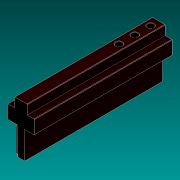
# Autodesk Inventor part: slider
Saved by Autodesk Inventor 2020.3 (Build 243373000, 373)
## iProperties
Created: 2020-05-25
Part Number: slider
Material: Generic
Document SubType Name: Modeling
Designer: Svend
Density: 1 g/cm^3
Appearance: Default
Author: Svend
Autodesk Inventor part; units mm, degrees
(part 1 of 2)
ref_plane "YZ Plane" through (0, 0, 0) normal (1, 0, 0) x (0, 1, 0)
ref_plane "XZ Plane" through (0, 0, 0) normal (0, 1, 0) x (-1, 0, 0)
ref_plane "XY Plane" through (0, 0, 0) normal (0, 0, 1) x (1, 0, 0)
sketch "Sketch1" plane through (0, 0, 0) normal (0, 0, 1) x (1, 0, 0)
  line L0 (-3.25, 4.8) -> (3.25, 4.8)
  line L1 (3.25, 4.8) -> (3.25, 0)
  line L2 (3.25, 0) -> (6.8, 0)
  line L3 (6.8, 0) -> (6.8, -7)
  line L4 (-3, -21) -> (-3, -7)
  line L5 (-6.8, -7) -> (-6.8, 0)
  line L6 (-6.8, 0) -> (-3.25, 0)
  line L7 (-3.25, 4.8) -> (-3.25, 0)
  line L8 (-3, -21) -> (3, -21)
  line L9 (6.8, -7) -> (3, -7)
  line L10 (-6.8, -7) -> (-3, -7)
  line L11 (3, -21) -> (3, -7)
  point P0 (0, 0)
  point P1 (0, 4.8)
  point P2 (0, -17.2)
  point P3 (0, -21)
  dimension "d0" = 6.5
  dimension "d1" = 4.8
  dimension "d6" = 14
  dimension "d7" = 7
  dimension "d8" = 6
  dimension "d9" = 13.6
  constraints: 24 end point, 5 perpendicular, 4 horizontal, 3 equal length, 3 point on line, 3 vertical alignment, 2 midpoint, 2 vertical
  measures "d0" distance between parallel lines of L7 L1
  measures "d1" distance between parallel lines of L2 L0
  measures "d6" distance of L4.start L4.end
  measures "d7" distance of L2.end L3.end
  measures "d8" distance between parallel lines of L4 L11
  measures "d9" distance between parallel lines of L5 L3
extrude "Extrusion1" add sketch "Sketch1" along normal mid plane 70
sketch "Sketch2" plane through (-3.25, 4.8, 35) normal (0, 1, 0) x (1, 0, 0)
  line L0 (0, 70) -> (0, 0) projected
  line L1 (6.5, 0) -> (0, 0) projected
  line L2 (6.5, 70) -> (6.5, 0) projected
  line L3 (0, 70) -> (6.5, 70) projected
  circle A0 centre (3.25, 49.7) radius 1.6
  circle A1 centre (3.25, 57.7) radius 1.6
  circle A2 centre (3.25, 65.7) radius 1.6
  point P0 (3.25, 35)
  dimension "d13" = 4.3
  dimension "d14" = 8
  dimension "d15" = 8
  dimension "d17" = 3.2
  constraints: 3 centre point, 3 coincident, 3 vertical alignment, 2 equal radius
  measures "d13" distance from line of point (3.25, 65.7) L3
  measures "d14" distance of point (3.25, 57.7) point (3.25, 65.7)
  measures "d15" distance of point (3.25, 57.7) point (3.25, 49.7)
  measures "d17" diameter of A0
extrude "Extrusion2" cut sketch "Sketch2" against normal blind 8.3 contours A0 | A1 | A2
sketch "Sketch3" plane through (0, 0, -35) normal (0, 0, -1) x (-1, 0, 0)
  line L0 (3, -21) -> (3, -7) projected
  line L1 (3, -7) -> (6.8, -7) projected
  line L2 (6.8, -7) -> (6.8, 0) projected
  line L3 (6.8, 0) -> (3.25, 0) projected
  line L4 (3.25, 0) -> (3.25, 4.8) projected
  line L5 (3.25, 4.8) -> (-3.25, 4.8) projected
  line L6 (-3.25, 4.8) -> (-3.25, 0) projected
  line L7 (-3.25, 0) -> (-6.8, 0) projected
  line L8 (-6.8, 0) -> (-6.8, -7) projected
  line L9 (-6.8, -7) -> (-3, -7) projected
  line L10 (-3, -7) -> (-3, -21) projected
  line L11 (-3, -21) -> (3, -21) projected
  line L12 (-1.6, -3.5) -> (1.6, -3.5) projected
  line L13 (-2.75, -1.5) -> (2.75, -1.5)
  line L14 (2.75, -1.5) -> (2.75, -5.5)
  line L15 (2.75, -5.5) -> (-2.75, -5.5)
  line L16 (-2.75, -5.5) -> (-2.75, -1.5)
  line L17 (-2.75, -1.5) -> (2.75, -5.5) construction
  line L18 (2.75, -1.5) -> (-2.75, -5.5) construction
  point P0 (0, 0)
  point P1 (0, -3.5)
  dimension "d21" = 5.5
  dimension "d22" = 4
  constraints: 12 end point, 3 midpoint, 2 parallel, 1 horizontal, 1 perpendicular
  measures "d21" distance of L14.end L15.end
  measures "d22" distance of L13.end L14.end
extrude "Extrusion3" cut sketch "Sketch3" against normal blind 25 contours L13 L14 L15 L16
chamfer "Chamfer1" distance 0.2 angle 45 8 edges at (6.8, 0, 0) (6.8, -7, 0) (3.25, 4.8, 0) (-3.25, 4.8, 0) (-6.8, 0, 0) (-6.8, -7, 0) (-3, -21, 0) (3, -21, 0)
chamfer "Chamfer2" distance 0.2 angle 45 3 edges at (-1.6, 4.8, -14.7) (-1.6, 4.8, -22.7) (-1.6, 4.8, -30.7)
chamfer "Chamfer3" distance 0.2 angle 45 16 edges at (4.925, 0, -35) (3.25, 2.3, -35) (0, 4.8, -35) (-3.25, 2.3, -35) (-4.925, 0, -35) (-6.8, -3.5, -35) (-4.8, -7, -35) (-3, -13.9, -35) (3, -13.9, -35) (4.8, -7, -35) (6.8, -3.5, -35) (0, -21, -35) (0, -5.5, -35) (-2.75, -3.5, -35) (0, -1.5, -35) (2.75, -3.5, -35)
sketch "Sketch4" plane through (0, 0, 35) normal (0, 0, 1) x (1, 0, 0)
  line L0 (3, -20.8) -> (2.8, -21) projected
  line L1 (3, -20.8) -> (3, -7) projected
  line L2 (3, -7) -> (6.6, -7) projected
  line L3 (6.8, -6.8) -> (6.6, -7) projected
  line L4 (6.8, -6.8) -> (6.8, -0.2) projected
  line L5 (6.6, 0) -> (6.8, -0.2) projected
  line L6 (6.6, 0) -> (3.25, 0) projected
  line L7 (3.25, 0) -> (3.25, 4.6) projected
  line L8 (3.05, 4.8) -> (3.25, 4.6) projected
  line L9 (3.05, 4.8) -> (-3.05, 4.8) projected
  line L10 (-3.25, 4.6) -> (-3.05, 4.8) projected
  line L11 (-3.25, 4.6) -> (-3.25, 0) projected
  line L12 (-3.25, 0) -> (-6.6, 0) projected
  line L13 (-6.8, -0.2) -> (-6.6, 0) projected
  line L14 (-6.8, -0.2) -> (-6.8, -6.8) projected
  line L15 (-6.6, -7) -> (-6.8, -6.8) projected
  line L16 (-6.6, -7) -> (-3, -7) projected
  line L17 (-3, -7) -> (-3, -20.8) projected
  line L18 (-2.8, -21) -> (-3, -20.8) projected
  line L19 (-2.8, -21) -> (2.8, -21) projected
  line L20 (-3, -7) -> (-1, -7)
  line L21 (-1, -7) -> (-1, -21)
  line L22 (2.8, -21) -> (-2.8, -21) projected
  point P0 (0, 0)
  dimension "d37" = 2
  constraints: 4 end point, 1 horizontal, 1 perpendicular, 1 point on line
  measures "d37" distance between parallel lines of L17 L21
extrude "Extrusion4" cut sketch "Sketch4" against normal through all contours L19 L18 L17 L20 L21
sketch "Sketch5" plane through (2.8, -21, -34.8) normal (0, -1, 0) x (1, 0, 0)
  line L0 (-4.55, 1.057) -> (-4.55, 2.6868)
  line L1 (-4.55, 2.6868) -> (-5.5, 2.6868)
  spline S0 degree 3 poles (-5.5, 2.6868) (-5.5115, 2.6868) (-5.5306, 2.6865) (-5.5581, 2.6853) (-5.5836, 2.6837) (-5.6121, 2.6814) (-5.6435, 2.6782) (-5.6779, 2.674) (-5.7151, 2.6686) (-5.7551, 2.6621) (-5.798, 2.6542) (-5.8437, 2.6449) (-5.8921, 2.6339) (-5.9432, 2.6213) (-5.9969, 2.6069) (-6.0532, 2.5906) (-6.1121, 2.5723) (-6.1734, 2.5518) (-6.2372, 2.5292) (-6.3033, 2.5041) (-6.3716, 2.4767) (-6.4422, 2.4467) (-6.5149, 2.4141) (-6.5897, 2.3787) (-6.6664, 2.3405) (-6.745, 2.2994) (-6.8162, 2.2604) (-6.8611, 2.2348) (-6.8794, 2.2242) knots 0 0 0 0 0.023552 0.038904 0.056302 0.075747 0.097239 0.120778 0.146364 0.173997 0.203676 0.235403 0.269176 0.304996 0.342863 0.382777 0.424738 0.468746 0.5148 0.562902 0.61305 0.665245 0.719487 0.775776 0.834112 0.894494 0.956924 1 1 1 1
  arc A0 (-6.8794, 2.2242) -> (-6.8794, 1.5196) centre (2.0124, 1.8719) ccw
  spline S1 degree 3 poles (-6.8794, 1.5196) (-6.8611, 1.509) (-6.8428, 1.4985) (-6.8244, 1.4882) (-6.7977, 1.4733) (-6.7709, 1.4585) (-6.744, 1.4441) (-6.7179, 1.4302) (-6.6917, 1.4165) (-6.6654, 1.403) (-6.6399, 1.39) (-6.6144, 1.3773) (-6.5887, 1.3649) (-6.5639, 1.3528) (-6.5389, 1.341) (-6.5139, 1.3295) (-6.4898, 1.3184) (-6.4655, 1.3075) (-6.4412, 1.2969) (-6.4178, 1.2867) (-6.3942, 1.2767) (-6.3706, 1.2669) (-6.3479, 1.2575) (-6.3251, 1.2484) (-6.3022, 1.2395) (-6.2803, 1.2309) (-6.2583, 1.2226) (-6.2362, 1.2145) (-6.215, 1.2067) (-6.1937, 1.1991) (-6.1724, 1.1918) (-6.152, 1.1848) (-6.1316, 1.178) (-6.1111, 1.1714) (-6.0915, 1.1651) (-6.0719, 1.1589) (-6.0522, 1.153) (-6.0335, 1.1474) (-6.0147, 1.142) (-5.9959, 1.1367) (-5.978, 1.1318) (-5.9601, 1.127) (-5.9422, 1.1224) (-5.9252, 1.118) (-5.9081, 1.1138) (-5.8911, 1.1098) (-5.875, 1.106) (-5.8588, 1.1023) (-5.8427, 1.0988) (-5.8275, 1.0956) (-5.8123, 1.0925) (-5.797, 1.0895) (-5.7827, 1.0867) (-5.7684, 1.0841) (-5.7541, 1.0816) (-5.7408, 1.0793) (-5.7274, 1.0771) (-5.7141, 1.0751) (-5.7017, 1.0732) (-5.6893, 1.0714) (-5.6768, 1.0698) (-5.6654, 1.0683) (-5.654, 1.0669) (-5.6425, 1.0656) (-5.6321, 1.0644) (-5.6216, 1.0633) (-5.6111, 1.0624) (-5.6016, 1.0615) (-5.5921, 1.0607) (-5.5826, 1.06) (-5.5741, 1.0594) (-5.5656, 1.0589) (-5.5571, 1.0585) (-5.5496, 1.0581) (-5.5421, 1.0578) (-5.5346, 1.0575) (-5.5231, 1.0572) (-5.5115, 1.057) (-5.5, 1.057) knots 0 0 0 0 0.043076 0.043076 0.043076 0.105506 0.105506 0.105506 0.165888 0.165888 0.165888 0.224224 0.224224 0.224224 0.280513 0.280513 0.280513 0.334755 0.334755 0.334755 0.38695 0.38695 0.38695 0.437099 0.437099 0.437099 0.4852 0.4852 0.4852 0.531254 0.531254 0.531254 0.575262 0.575262 0.575262 0.617223 0.617223 0.617223 0.657137 0.657137 0.657137 0.695004 0.695004 0.695004 0.730824 0.730824 0.730824 0.764598 0.764598 0.764598 0.796324 0.796324 0.796324 0.826004 0.826004 0.826004 0.853636 0.853636 0.853636 0.879222 0.879222 0.879222 0.902761 0.902761 0.902761 0.924253 0.924253 0.924253 0.943699 0.943699 0.943699 0.961097 0.961097 0.961097 0.976448 0.976448 0.976448 1 1 1 1
  line L2 (-5.5, 1.057) -> (-4.55, 1.057)
  line L3 (-4.55, 4.193) -> (-4.55, 5.8228)
  line L4 (-4.55, 5.8228) -> (-5.5, 5.8228)
  spline S2 degree 3 poles (-5.5, 5.8228) (-5.5115, 5.8228) (-5.5306, 5.8225) (-5.5581, 5.8213) (-5.5836, 5.8197) (-5.6121, 5.8174) (-5.6435, 5.8142) (-5.6779, 5.81) (-5.7151, 5.8046) (-5.7551, 5.7981) (-5.798, 5.7902) (-5.8437, 5.7809) (-5.8921, 5.7699) (-5.9432, 5.7573) (-5.9969, 5.7429) (-6.0532, 5.7266) (-6.1121, 5.7083) (-6.1734, 5.6878) (-6.2372, 5.6652) (-6.3033, 5.6401) (-6.3716, 5.6127) (-6.4422, 5.5827) (-6.5149, 5.5501) (-6.5897, 5.5147) (-6.6664, 5.4765) (-6.745, 5.4354) (-6.8162, 5.3964) (-6.8611, 5.3708) (-6.8794, 5.3602) knots 0 0 0 0 0.023552 0.038904 0.056302 0.075747 0.097239 0.120778 0.146364 0.173997 0.203676 0.235403 0.269176 0.304996 0.342863 0.382777 0.424738 0.468746 0.5148 0.562902 0.61305 0.665245 0.719487 0.775776 0.834112 0.894494 0.956924 1 1 1 1
  arc A1 (-6.8794, 5.3602) -> (-6.8794, 4.6556) centre (2.0124, 5.0079) ccw
  spline S3 degree 3 poles (-6.8794, 4.6556) (-6.8611, 4.645) (-6.8428, 4.6345) (-6.8244, 4.6242) (-6.7977, 4.6093) (-6.7709, 4.5945) (-6.744, 4.5801) (-6.7179, 4.5662) (-6.6917, 4.5525) (-6.6654, 4.539) (-6.6399, 4.526) (-6.6144, 4.5133) (-6.5887, 4.5009) (-6.5639, 4.4888) (-6.5389, 4.477) (-6.5139, 4.4655) (-6.4898, 4.4544) (-6.4655, 4.4435) (-6.4412, 4.4329) (-6.4178, 4.4227) (-6.3942, 4.4127) (-6.3706, 4.4029) (-6.3479, 4.3935) (-6.3251, 4.3844) (-6.3022, 4.3755) (-6.2803, 4.3669) (-6.2583, 4.3586) (-6.2362, 4.3505) (-6.215, 4.3427) (-6.1937, 4.3351) (-6.1724, 4.3278) (-6.152, 4.3208) (-6.1316, 4.314) (-6.1111, 4.3074) (-6.0915, 4.3011) (-6.0719, 4.2949) (-6.0522, 4.289) (-6.0335, 4.2834) (-6.0147, 4.278) (-5.9959, 4.2727) (-5.978, 4.2678) (-5.9601, 4.263) (-5.9422, 4.2584) (-5.9252, 4.254) (-5.9081, 4.2498) (-5.8911, 4.2458) (-5.875, 4.242) (-5.8588, 4.2383) (-5.8427, 4.2348) (-5.8275, 4.2316) (-5.8123, 4.2285) (-5.797, 4.2255) (-5.7827, 4.2227) (-5.7684, 4.2201) (-5.7541, 4.2176) (-5.7408, 4.2153) (-5.7274, 4.2131) (-5.7141, 4.2111) (-5.7017, 4.2092) (-5.6893, 4.2074) (-5.6768, 4.2058) (-5.6654, 4.2043) (-5.654, 4.2029) (-5.6425, 4.2016) (-5.6321, 4.2004) (-5.6216, 4.1993) (-5.6111, 4.1984) (-5.6016, 4.1975) (-5.5921, 4.1967) (-5.5826, 4.196) (-5.5741, 4.1954) (-5.5656, 4.1949) (-5.5571, 4.1945) (-5.5496, 4.1941) (-5.5421, 4.1938) (-5.5346, 4.1935) (-5.5231, 4.1932) (-5.5115, 4.193) (-5.5, 4.193) knots 0 0 0 0 0.043076 0.043076 0.043076 0.105506 0.105506 0.105506 0.165888 0.165888 0.165888 0.224224 0.224224 0.224224 0.280513 0.280513 0.280513 0.334755 0.334755 0.334755 0.38695 0.38695 0.38695 0.437099 0.437099 0.437099 0.4852 0.4852 0.4852 0.531254 0.531254 0.531254 0.575262 0.575262 0.575262 0.617223 0.617223 0.617223 0.657137 0.657137 0.657137 0.695004 0.695004 0.695004 0.730824 0.730824 0.730824 0.764598 0.764598 0.764598 0.796324 0.796324 0.796324 0.826004 0.826004 0.826004 0.853636 0.853636 0.853636 0.879222 0.879222 0.879222 0.902761 0.902761 0.902761 0.924253 0.924253 0.924253 0.943699 0.943699 0.943699 0.961097 0.961097 0.961097 0.976448 0.976448 0.976448 1 1 1 1
  line L5 (-5.5, 4.193) -> (-4.55, 4.193)
  line L6 (-4.55, 7.329) -> (-4.55, 8.9588)
  line L7 (-4.55, 8.9588) -> (-5.5, 8.9588)
  spline S4 degree 3 poles (-5.5, 8.9588) (-5.5115, 8.9588) (-5.5306, 8.9585) (-5.5581, 8.9573) (-5.5836, 8.9557) (-5.6121, 8.9534) (-5.6435, 8.9502) (-5.6779, 8.946) (-5.7151, 8.9406) (-5.7551, 8.9341) (-5.798, 8.9262) (-5.8437, 8.9169) (-5.8921, 8.9059) (-5.9432, 8.8933) (-5.9969, 8.8789) (-6.0532, 8.8626) (-6.1121, 8.8443) (-6.1734, 8.8238) (-6.2372, 8.8012) (-6.3033, 8.7761) (-6.3716, 8.7487) (-6.4422, 8.7187) (-6.5149, 8.6861) (-6.5897, 8.6507) (-6.6664, 8.6125) (-6.745, 8.5714) (-6.8162, 8.5324) (-6.8611, 8.5068) (-6.8794, 8.4962) knots 0 0 0 0 0.023552 0.038904 0.056302 0.075747 0.097239 0.120778 0.146364 0.173997 0.203676 0.235403 0.269176 0.304996 0.342863 0.382777 0.424738 0.468746 0.5148 0.562902 0.61305 0.665245 0.719487 0.775776 0.834112 0.894494 0.956924 1 1 1 1
  arc A2 (-6.8794, 8.4962) -> (-6.8794, 7.7916) centre (2.0124, 8.1439) ccw
  spline S5 degree 3 poles (-6.8794, 7.7916) (-6.8611, 7.781) (-6.8428, 7.7705) (-6.8244, 7.7602) (-6.7977, 7.7453) (-6.7709, 7.7305) (-6.744, 7.7161) (-6.7179, 7.7022) (-6.6917, 7.6885) (-6.6654, 7.675) (-6.6399, 7.662) (-6.6144, 7.6493) (-6.5887, 7.6369) (-6.5639, 7.6248) (-6.5389, 7.613) (-6.5139, 7.6015) (-6.4898, 7.5904) (-6.4655, 7.5795) (-6.4412, 7.5689) (-6.4178, 7.5587) (-6.3942, 7.5487) (-6.3706, 7.5389) (-6.3479, 7.5295) (-6.3251, 7.5204) (-6.3022, 7.5115) (-6.2803, 7.5029) (-6.2583, 7.4946) (-6.2362, 7.4865) (-6.215, 7.4787) (-6.1937, 7.4711) (-6.1724, 7.4638) (-6.152, 7.4568) (-6.1316, 7.45) (-6.1111, 7.4434) (-6.0915, 7.4371) (-6.0719, 7.4309) (-6.0522, 7.425) (-6.0335, 7.4194) (-6.0147, 7.414) (-5.9959, 7.4087) (-5.978, 7.4038) (-5.9601, 7.399) (-5.9422, 7.3944) (-5.9252, 7.39) (-5.9081, 7.3858) (-5.8911, 7.3818) (-5.875, 7.378) (-5.8588, 7.3743) (-5.8427, 7.3708) (-5.8275, 7.3676) (-5.8123, 7.3645) (-5.797, 7.3615) (-5.7827, 7.3587) (-5.7684, 7.3561) (-5.7541, 7.3536) (-5.7408, 7.3513) (-5.7274, 7.3491) (-5.7141, 7.3471) (-5.7017, 7.3452) (-5.6893, 7.3434) (-5.6768, 7.3418) (-5.6654, 7.3403) (-5.654, 7.3389) (-5.6425, 7.3376) (-5.6321, 7.3364) (-5.6216, 7.3353) (-5.6111, 7.3344) (-5.6016, 7.3335) (-5.5921, 7.3327) (-5.5826, 7.332) (-5.5741, 7.3314) (-5.5656, 7.3309) (-5.5571, 7.3305) (-5.5496, 7.3301) (-5.5421, 7.3298) (-5.5346, 7.3295) (-5.5231, 7.3292) (-5.5115, 7.329) (-5.5, 7.329) knots 0 0 0 0 0.043076 0.043076 0.043076 0.105506 0.105506 0.105506 0.165888 0.165888 0.165888 0.224224 0.224224 0.224224 0.280513 0.280513 0.280513 0.334755 0.334755 0.334755 0.38695 0.38695 0.38695 0.437099 0.437099 0.437099 0.4852 0.4852 0.4852 0.531254 0.531254 0.531254 0.575262 0.575262 0.575262 0.617223 0.617223 0.617223 0.657137 0.657137 0.657137 0.695004 0.695004 0.695004 0.730824 0.730824 0.730824 0.764598 0.764598 0.764598 0.796324 0.796324 0.796324 0.826004 0.826004 0.826004 0.853636 0.853636 0.853636 0.879222 0.879222 0.879222 0.902761 0.902761 0.902761 0.924253 0.924253 0.924253 0.943699 0.943699 0.943699 0.961097 0.961097 0.961097 0.976448 0.976448 0.976448 1 1 1 1
  line L8 (-5.5, 7.329) -> (-4.55, 7.329)
  line L9 (-4.55, 10.465) -> (-4.55, 12.0948)
  line L10 (-4.55, 12.0948) -> (-5.5, 12.0948)
  spline S6 degree 3 poles (-5.5, 12.0948) (-5.5115, 12.0948) (-5.5306, 12.0945) (-5.5581, 12.0933) (-5.5836, 12.0917) (-5.6121, 12.0894) (-5.6435, 12.0862) (-5.6779, 12.082) (-5.7151, 12.0766) (-5.7551, 12.0701) (-5.798, 12.0622) (-5.8437, 12.0529) (-5.8921, 12.0419) (-5.9432, 12.0293) (-5.9969, 12.0149) (-6.0532, 11.9986) (-6.1121, 11.9803) (-6.1734, 11.9598) (-6.2372, 11.9372) (-6.3033, 11.9121) (-6.3716, 11.8847) (-6.4422, 11.8547) (-6.5149, 11.8221) (-6.5897, 11.7867) (-6.6664, 11.7485) (-6.745, 11.7074) (-6.8162, 11.6684) (-6.8611, 11.6428) (-6.8794, 11.6322) knots 0 0 0 0 0.023552 0.038904 0.056302 0.075747 0.097239 0.120778 0.146364 0.173997 0.203676 0.235403 0.269176 0.304996 0.342863 0.382777 0.424738 0.468746 0.5148 0.562902 0.61305 0.665245 0.719487 0.775776 0.834112 0.894494 0.956924 1 1 1 1
  arc A3 (-6.8794, 11.6322) -> (-6.8794, 10.9276) centre (2.0124, 11.2799) ccw
  spline S7 degree 3 poles (-6.8794, 10.9276) (-6.8611, 10.917) (-6.8428, 10.9065) (-6.8244, 10.8962) (-6.7977, 10.8813) (-6.7709, 10.8665) (-6.744, 10.8521) (-6.7179, 10.8382) (-6.6917, 10.8245) (-6.6654, 10.811) (-6.6399, 10.798) (-6.6144, 10.7853) (-6.5887, 10.7729) (-6.5639, 10.7608) (-6.5389, 10.749) (-6.5139, 10.7375) (-6.4898, 10.7264) (-6.4655, 10.7155) (-6.4412, 10.7049) (-6.4178, 10.6947) (-6.3942, 10.6847) (-6.3706, 10.6749) (-6.3479, 10.6655) (-6.3251, 10.6564) (-6.3022, 10.6475) (-6.2803, 10.6389) (-6.2583, 10.6306) (-6.2362, 10.6225) (-6.215, 10.6147) (-6.1937, 10.6071) (-6.1724, 10.5998) (-6.152, 10.5928) (-6.1316, 10.586) (-6.1111, 10.5794) (-6.0915, 10.5731) (-6.0719, 10.5669) (-6.0522, 10.561) (-6.0335, 10.5554) (-6.0147, 10.55) (-5.9959, 10.5447) (-5.978, 10.5398) (-5.9601, 10.535) (-5.9422, 10.5304) (-5.9252, 10.526) (-5.9081, 10.5218) (-5.8911, 10.5178) (-5.875, 10.514) (-5.8588, 10.5103) (-5.8427, 10.5068) (-5.8275, 10.5036) (-5.8123, 10.5005) (-5.797, 10.4975) (-5.7827, 10.4947) (-5.7684, 10.4921) (-5.7541, 10.4896) (-5.7408, 10.4873) (-5.7274, 10.4851) (-5.7141, 10.4831) (-5.7017, 10.4812) (-5.6893, 10.4794) (-5.6768, 10.4778) (-5.6654, 10.4763) (-5.654, 10.4749) (-5.6425, 10.4736) (-5.6321, 10.4724) (-5.6216, 10.4713) (-5.6111, 10.4704) (-5.6016, 10.4695) (-5.5921, 10.4687) (-5.5826, 10.468) (-5.5741, 10.4674) (-5.5656, 10.4669) (-5.5571, 10.4665) (-5.5496, 10.4661) (-5.5421, 10.4658) (-5.5346, 10.4655) (-5.5231, 10.4652) (-5.5115, 10.465) (-5.5, 10.465) knots 0 0 0 0 0.043076 0.043076 0.043076 0.105506 0.105506 0.105506 0.165888 0.165888 0.165888 0.224224 0.224224 0.224224 0.280513 0.280513 0.280513 0.334755 0.334755 0.334755 0.38695 0.38695 0.38695 0.437099 0.437099 0.437099 0.4852 0.4852 0.4852 0.531254 0.531254 0.531254 0.575262 0.575262 0.575262 0.617223 0.617223 0.617223 0.657137 0.657137 0.657137 0.695004 0.695004 0.695004 0.730824 0.730824 0.730824 0.764598 0.764598 0.764598 0.796324 0.796324 0.796324 0.826004 0.826004 0.826004 0.853636 0.853636 0.853636 0.879222 0.879222 0.879222 0.902761 0.902761 0.902761 0.924253 0.924253 0.924253 0.943699 0.943699 0.943699 0.961097 0.961097 0.961097 0.976448 0.976448 0.976448 1 1 1 1
  line L11 (-5.5, 10.465) -> (-4.55, 10.465)
  line L12 (-4.55, 13.601) -> (-4.55, 15.2308)
  line L13 (-4.55, 15.2308) -> (-5.5, 15.2308)
  spline S8 degree 3 poles (-5.5, 15.2308) (-5.5115, 15.2308) (-5.5306, 15.2305) (-5.5581, 15.2293) (-5.5836, 15.2277) (-5.6121, 15.2254) (-5.6435, 15.2222) (-5.6779, 15.218) (-5.7151, 15.2126) (-5.7551, 15.2061) (-5.798, 15.1982) (-5.8437, 15.1889) (-5.8921, 15.1779) (-5.9432, 15.1653) (-5.9969, 15.1509) (-6.0532, 15.1346) (-6.1121, 15.1163) (-6.1734, 15.0958) (-6.2372, 15.0732) (-6.3033, 15.0481) (-6.3716, 15.0207) (-6.4422, 14.9907) (-6.5149, 14.9581) (-6.5897, 14.9227) (-6.6664, 14.8845) (-6.745, 14.8434) (-6.8162, 14.8044) (-6.8611, 14.7788) (-6.8794, 14.7682) knots 0 0 0 0 0.023552 0.038904 0.056302 0.075747 0.097239 0.120778 0.146364 0.173997 0.203676 0.235403 0.269176 0.304996 0.342863 0.382777 0.424738 0.468746 0.5148 0.562902 0.61305 0.665245 0.719487 0.775776 0.834112 0.894494 0.956924 1 1 1 1
  arc A4 (-6.8794, 14.7682) -> (-6.8794, 14.0636) centre (2.0124, 14.4159) ccw
  spline S9 degree 3 poles (-6.8794, 14.0636) (-6.8611, 14.053) (-6.8428, 14.0425) (-6.8244, 14.0322) (-6.7977, 14.0173) (-6.7709, 14.0025) (-6.744, 13.9881) (-6.7179, 13.9742) (-6.6917, 13.9605) (-6.6654, 13.947) (-6.6399, 13.934) (-6.6144, 13.9213) (-6.5887, 13.9089) (-6.5639, 13.8968) (-6.5389, 13.885) (-6.5139, 13.8735) (-6.4898, 13.8624) (-6.4655, 13.8515) (-6.4412, 13.8409) (-6.4178, 13.8307) (-6.3942, 13.8207) (-6.3706, 13.8109) (-6.3479, 13.8015) (-6.3251, 13.7924) (-6.3022, 13.7835) (-6.2803, 13.7749) (-6.2583, 13.7666) (-6.2362, 13.7585) (-6.215, 13.7507) (-6.1937, 13.7431) (-6.1724, 13.7358) (-6.152, 13.7288) (-6.1316, 13.722) (-6.1111, 13.7154) (-6.0915, 13.7091) (-6.0719, 13.7029) (-6.0522, 13.697) (-6.0335, 13.6914) (-6.0147, 13.686) (-5.9959, 13.6807) (-5.978, 13.6758) (-5.9601, 13.671) (-5.9422, 13.6664) (-5.9252, 13.662) (-5.9081, 13.6578) (-5.8911, 13.6538) (-5.875, 13.65) (-5.8588, 13.6463) (-5.8427, 13.6428) (-5.8275, 13.6396) (-5.8123, 13.6365) (-5.797, 13.6335) (-5.7827, 13.6307) (-5.7684, 13.6281) (-5.7541, 13.6256) (-5.7408, 13.6233) (-5.7274, 13.6211) (-5.7141, 13.6191) (-5.7017, 13.6172) (-5.6893, 13.6154) (-5.6768, 13.6138) (-5.6654, 13.6123) (-5.654, 13.6109) (-5.6425, 13.6096) (-5.6321, 13.6084) (-5.6216, 13.6073) (-5.6111, 13.6064) (-5.6016, 13.6055) (-5.5921, 13.6047) (-5.5826, 13.604) (-5.5741, 13.6034) (-5.5656, 13.6029) (-5.5571, 13.6025) (-5.5496, 13.6021) (-5.5421, 13.6018) (-5.5346, 13.6015) (-5.5231, 13.6012) (-5.5115, 13.601) (-5.5, 13.601) knots 0 0 0 0 0.043076 0.043076 0.043076 0.105506 0.105506 0.105506 0.165888 0.165888 0.165888 0.224224 0.224224 0.224224 0.280513 0.280513 0.280513 0.334755 0.334755 0.334755 0.38695 0.38695 0.38695 0.437099 0.437099 0.437099 0.4852 0.4852 0.4852 0.531254 0.531254 0.531254 0.575262 0.575262 0.575262 0.617223 0.617223 0.617223 0.657137 0.657137 0.657137 0.695004 0.695004 0.695004 0.730824 0.730824 0.730824 0.764598 0.764598 0.764598 0.796324 0.796324 0.796324 0.826004 0.826004 0.826004 0.853636 0.853636 0.853636 0.879222 0.879222 0.879222 0.902761 0.902761 0.902761 0.924253 0.924253 0.924253 0.943699 0.943699 0.943699 0.961097 0.961097 0.961097 0.976448 0.976448 0.976448 1 1 1 1
  line L14 (-5.5, 13.601) -> (-4.55, 13.601)
  line L15 (-4.55, 16.737) -> (-4.55, 18.3668)
  line L16 (-4.55, 18.3668) -> (-5.5, 18.3668)
  spline S10 degree 3 poles (-5.5, 18.3668) (-5.5115, 18.3668) (-5.5306, 18.3665) (-5.5581, 18.3653) (-5.5836, 18.3637) (-5.6121, 18.3614) (-5.6435, 18.3582) (-5.6779, 18.354) (-5.7151, 18.3486) (-5.7551, 18.3421) (-5.798, 18.3342) (-5.8437, 18.3249) (-5.8921, 18.3139) (-5.9432, 18.3013) (-5.9969, 18.2869) (-6.0532, 18.2706) (-6.1121, 18.2523) (-6.1734, 18.2318) (-6.2372, 18.2092) (-6.3033, 18.1841) (-6.3716, 18.1567) (-6.4422, 18.1267) (-6.5149, 18.0941) (-6.5897, 18.0587) (-6.6664, 18.0205) (-6.745, 17.9794) (-6.8162, 17.9404) (-6.8611, 17.9148) (-6.8794, 17.9042) knots 0 0 0 0 0.023552 0.038904 0.056302 0.075747 0.097239 0.120778 0.146364 0.173997 0.203676 0.235403 0.269176 0.304996 0.342863 0.382777 0.424738 0.468746 0.5148 0.562902 0.61305 0.665245 0.719487 0.775776 0.834112 0.894494 0.956924 1 1 1 1
  arc A5 (-6.8794, 17.9042) -> (-6.8794, 17.1996) centre (2.0124, 17.5519) ccw
  spline S11 degree 3 poles (-6.8794, 17.1996) (-6.8611, 17.189) (-6.8428, 17.1785) (-6.8244, 17.1682) (-6.7977, 17.1533) (-6.7709, 17.1385) (-6.744, 17.1241) (-6.7179, 17.1102) (-6.6917, 17.0965) (-6.6654, 17.083) (-6.6399, 17.07) (-6.6144, 17.0573) (-6.5887, 17.0449) (-6.5639, 17.0328) (-6.5389, 17.021) (-6.5139, 17.0095) (-6.4898, 16.9984) (-6.4655, 16.9875) (-6.4412, 16.9769) (-6.4178, 16.9667) (-6.3942, 16.9567) (-6.3706, 16.9469) (-6.3479, 16.9375) (-6.3251, 16.9284) (-6.3022, 16.9195) (-6.2803, 16.9109) (-6.2583, 16.9026) (-6.2362, 16.8945) (-6.215, 16.8867) (-6.1937, 16.8791) (-6.1724, 16.8718) (-6.152, 16.8648) (-6.1316, 16.858) (-6.1111, 16.8514) (-6.0915, 16.8451) (-6.0719, 16.8389) (-6.0522, 16.833) (-6.0335, 16.8274) (-6.0147, 16.822) (-5.9959, 16.8167) (-5.978, 16.8118) (-5.9601, 16.807) (-5.9422, 16.8024) (-5.9252, 16.798) (-5.9081, 16.7938) (-5.8911, 16.7898) (-5.875, 16.786) (-5.8588, 16.7823) (-5.8427, 16.7788) (-5.8275, 16.7756) (-5.8123, 16.7725) (-5.797, 16.7695) (-5.7827, 16.7667) (-5.7684, 16.7641) (-5.7541, 16.7616) (-5.7408, 16.7593) (-5.7274, 16.7571) (-5.7141, 16.7551) (-5.7017, 16.7532) (-5.6893, 16.7514) (-5.6768, 16.7498) (-5.6654, 16.7483) (-5.654, 16.7469) (-5.6425, 16.7456) (-5.6321, 16.7444) (-5.6216, 16.7433) (-5.6111, 16.7424) (-5.6016, 16.7415) (-5.5921, 16.7407) (-5.5826, 16.74) (-5.5741, 16.7394) (-5.5656, 16.7389) (-5.5571, 16.7385) (-5.5496, 16.7381) (-5.5421, 16.7378) (-5.5346, 16.7375) (-5.5231, 16.7372) (-5.5115, 16.737) (-5.5, 16.737) knots 0 0 0 0 0.043076 0.043076 0.043076 0.105506 0.105506 0.105506 0.165888 0.165888 0.165888 0.224224 0.224224 0.224224 0.280513 0.280513 0.280513 0.334755 0.334755 0.334755 0.38695 0.38695 0.38695 0.437099 0.437099 0.437099 0.4852 0.4852 0.4852 0.531254 0.531254 0.531254 0.575262 0.575262 0.575262 0.617223 0.617223 0.617223 0.657137 0.657137 0.657137 0.695004 0.695004 0.695004 0.730824 0.730824 0.730824 0.764598 0.764598 0.764598 0.796324 0.796324 0.796324 0.826004 0.826004 0.826004 0.853636 0.853636 0.853636 0.879222 0.879222 0.879222 0.902761 0.902761 0.902761 0.924253 0.924253 0.924253 0.943699 0.943699 0.943699 0.961097 0.961097 0.961097 0.976448 0.976448 0.976448 1 1 1 1
  line L17 (-5.5, 16.737) -> (-4.55, 16.737)
  line L18 (-4.55, 19.873) -> (-4.55, 21.5028)
  line L19 (-4.55, 21.5028) -> (-5.5, 21.5028)
  spline S12 degree 3 poles (-5.5, 21.5028) (-5.5115, 21.5028) (-5.5306, 21.5025) (-5.5581, 21.5013) (-5.5836, 21.4997) (-5.6121, 21.4974) (-5.6435, 21.4942) (-5.6779, 21.49) (-5.7151, 21.4846) (-5.7551, 21.4781) (-5.798, 21.4702) (-5.8437, 21.4609) (-5.8921, 21.4499) (-5.9432, 21.4373) (-5.9969, 21.4229) (-6.0532, 21.4066) (-6.1121, 21.3883) (-6.1734, 21.3678) (-6.2372, 21.3452) (-6.3033, 21.3201) (-6.3716, 21.2927) (-6.4422, 21.2627) (-6.5149, 21.2301) (-6.5897, 21.1947) (-6.6664, 21.1565) (-6.745, 21.1154) (-6.8162, 21.0764) (-6.8611, 21.0508) (-6.8794, 21.0402) knots 0 0 0 0 0.023552 0.038904 0.056302 0.075747 0.097239 0.120778 0.146364 0.173997 0.203676 0.235403 0.269176 0.304996 0.342863 0.382777 0.424738 0.468746 0.5148 0.562902 0.61305 0.665245 0.719487 0.775776 0.834112 0.894494 0.956924 1 1 1 1
  arc A6 (-6.8794, 21.0402) -> (-6.8794, 20.3356) centre (2.0124, 20.6879) ccw
  spline S13 degree 3 poles (-6.8794, 20.3356) (-6.8611, 20.325) (-6.8428, 20.3145) (-6.8244, 20.3042) (-6.7977, 20.2893) (-6.7709, 20.2745) (-6.744, 20.2601) (-6.7179, 20.2462) (-6.6917, 20.2325) (-6.6654, 20.219) (-6.6399, 20.206) (-6.6144, 20.1933) (-6.5887, 20.1809) (-6.5639, 20.1688) (-6.5389, 20.157) (-6.5139, 20.1455) (-6.4898, 20.1344) (-6.4655, 20.1235) (-6.4412, 20.1129) (-6.4178, 20.1027) (-6.3942, 20.0927) (-6.3706, 20.0829) (-6.3479, 20.0735) (-6.3251, 20.0644) (-6.3022, 20.0555) (-6.2803, 20.0469) (-6.2583, 20.0386) (-6.2362, 20.0305) (-6.215, 20.0227) (-6.1937, 20.0151) (-6.1724, 20.0078) (-6.152, 20.0008) (-6.1316, 19.994) (-6.1111, 19.9874) (-6.0915, 19.9811) (-6.0719, 19.9749) (-6.0522, 19.969) (-6.0335, 19.9634) (-6.0147, 19.958) (-5.9959, 19.9527) (-5.978, 19.9478) (-5.9601, 19.943) (-5.9422, 19.9384) (-5.9252, 19.934) (-5.9081, 19.9298) (-5.8911, 19.9258) (-5.875, 19.922) (-5.8588, 19.9183) (-5.8427, 19.9148) (-5.8275, 19.9116) (-5.8123, 19.9085) (-5.797, 19.9055) (-5.7827, 19.9027) (-5.7684, 19.9001) (-5.7541, 19.8976) (-5.7408, 19.8953) (-5.7274, 19.8931) (-5.7141, 19.8911) (-5.7017, 19.8892) (-5.6893, 19.8874) (-5.6768, 19.8858) (-5.6654, 19.8843) (-5.654, 19.8829) (-5.6425, 19.8816) (-5.6321, 19.8804) (-5.6216, 19.8793) (-5.6111, 19.8784) (-5.6016, 19.8775) (-5.5921, 19.8767) (-5.5826, 19.876) (-5.5741, 19.8754) (-5.5656, 19.8749) (-5.5571, 19.8745) (-5.5496, 19.8741) (-5.5421, 19.8738) (-5.5346, 19.8735) (-5.5231, 19.8732) (-5.5115, 19.873) (-5.5, 19.873) knots 0 0 0 0 0.043076 0.043076 0.043076 0.105506 0.105506 0.105506 0.165888 0.165888 0.165888 0.224224 0.224224 0.224224 0.280513 0.280513 0.280513 0.334755 0.334755 0.334755 0.38695 0.38695 0.38695 0.437099 0.437099 0.437099 0.4852 0.4852 0.4852 0.531254 0.531254 0.531254 0.575262 0.575262 0.575262 0.617223 0.617223 0.617223 0.657137 0.657137 0.657137 0.695004 0.695004 0.695004 0.730824 0.730824 0.730824 0.764598 0.764598 0.764598 0.796324 0.796324 0.796324 0.826004 0.826004 0.826004 0.853636 0.853636 0.853636 0.879222 0.879222 0.879222 0.902761 0.902761 0.902761 0.924253 0.924253 0.924253 0.943699 0.943699 0.943699 0.961097 0.961097 0.961097 0.976448 0.976448 0.976448 1 1 1 1
  line L20 (-5.5, 19.873) -> (-4.55, 19.873)
  line L21 (-4.55, 23.009) -> (-4.55, 24.6388)
  line L22 (-4.55, 24.6388) -> (-5.5, 24.6388)
  spline S14 degree 3 poles (-5.5, 24.6388) (-5.5115, 24.6388) (-5.5306, 24.6385) (-5.5581, 24.6373) (-5.5836, 24.6357) (-5.6121, 24.6334) (-5.6435, 24.6302) (-5.6779, 24.626) (-5.7151, 24.6206) (-5.7551, 24.6141) (-5.798, 24.6062) (-5.8437, 24.5969) (-5.8921, 24.5859) (-5.9432, 24.5733) (-5.9969, 24.5589) (-6.0532, 24.5426) (-6.1121, 24.5243) (-6.1734, 24.5038) (-6.2372, 24.4812) (-6.3033, 24.4561) (-6.3716, 24.4287) (-6.4422, 24.3987) (-6.5149, 24.3661) (-6.5897, 24.3307) (-6.6664, 24.2925) (-6.745, 24.2514) (-6.8162, 24.2124) (-6.8611, 24.1868) (-6.8794, 24.1762) knots 0 0 0 0 0.023552 0.038904 0.056302 0.075747 0.097239 0.120778 0.146364 0.173997 0.203676 0.235403 0.269176 0.304996 0.342863 0.382777 0.424738 0.468746 0.5148 0.562902 0.61305 0.665245 0.719487 0.775776 0.834112 0.894494 0.956924 1 1 1 1
  arc A7 (-6.8794, 24.1762) -> (-6.8794, 23.4716) centre (2.0124, 23.8239) ccw
  spline S15 degree 3 poles (-6.8794, 23.4716) (-6.8611, 23.461) (-6.8428, 23.4505) (-6.8244, 23.4402) (-6.7977, 23.4253) (-6.7709, 23.4105) (-6.744, 23.3961) (-6.7179, 23.3822) (-6.6917, 23.3685) (-6.6654, 23.355) (-6.6399, 23.342) (-6.6144, 23.3293) (-6.5887, 23.3169) (-6.5639, 23.3048) (-6.5389, 23.293) (-6.5139, 23.2815) (-6.4898, 23.2704) (-6.4655, 23.2595) (-6.4412, 23.2489) (-6.4178, 23.2387) (-6.3942, 23.2287) (-6.3706, 23.2189) (-6.3479, 23.2095) (-6.3251, 23.2004) (-6.3022, 23.1915) (-6.2803, 23.1829) (-6.2583, 23.1746) (-6.2362, 23.1665) (-6.215, 23.1587) (-6.1937, 23.1511) (-6.1724, 23.1438) (-6.152, 23.1368) (-6.1316, 23.13) (-6.1111, 23.1234) (-6.0915, 23.1171) (-6.0719, 23.1109) (-6.0522, 23.105) (-6.0335, 23.0994) (-6.0147, 23.094) (-5.9959, 23.0887) (-5.978, 23.0838) (-5.9601, 23.079) (-5.9422, 23.0744) (-5.9252, 23.07) (-5.9081, 23.0658) (-5.8911, 23.0618) (-5.875, 23.058) (-5.8588, 23.0543) (-5.8427, 23.0508) (-5.8275, 23.0476) (-5.8123, 23.0445) (-5.797, 23.0415) (-5.7827, 23.0387) (-5.7684, 23.0361) (-5.7541, 23.0336) (-5.7408, 23.0313) (-5.7274, 23.0291) (-5.7141, 23.0271) (-5.7017, 23.0252) (-5.6893, 23.0234) (-5.6768, 23.0218) (-5.6654, 23.0203) (-5.654, 23.0189) (-5.6425, 23.0176) (-5.6321, 23.0164) (-5.6216, 23.0153) (-5.6111, 23.0144) (-5.6016, 23.0135) (-5.5921, 23.0127) (-5.5826, 23.012) (-5.5741, 23.0114) (-5.5656, 23.0109) (-5.5571, 23.0105) (-5.5496, 23.0101) (-5.5421, 23.0098) (-5.5346, 23.0095) (-5.5231, 23.0092) (-5.5115, 23.009) (-5.5, 23.009) knots 0 0 0 0 0.043076 0.043076 0.043076 0.105506 0.105506 0.105506 0.165888 0.165888 0.165888 0.224224 0.224224 0.224224 0.280513 0.280513 0.280513 0.334755 0.334755 0.334755 0.38695 0.38695 0.38695 0.437099 0.437099 0.437099 0.4852 0.4852 0.4852 0.531254 0.531254 0.531254 0.575262 0.575262 0.575262 0.617223 0.617223 0.617223 0.657137 0.657137 0.657137 0.695004 0.695004 0.695004 0.730824 0.730824 0.730824 0.764598 0.764598 0.764598 0.796324 0.796324 0.796324 0.826004 0.826004 0.826004 0.853636 0.853636 0.853636 0.879222 0.879222 0.879222 0.902761 0.902761 0.902761 0.924253 0.924253 0.924253 0.943699 0.943699 0.943699 0.961097 0.961097 0.961097 0.976448 0.976448 0.976448 1 1 1 1
  line L23 (-5.5, 23.009) -> (-4.55, 23.009)
  line L24 (-4.55, 26.145) -> (-4.55, 27.7748)
  line L25 (-4.55, 27.7748) -> (-5.5, 27.7748)
  spline S16 degree 3 poles (-5.5, 27.7748) (-5.5115, 27.7748) (-5.5306, 27.7745) (-5.5581, 27.7733) (-5.5836, 27.7717) (-5.6121, 27.7694) (-5.6435, 27.7662) (-5.6779, 27.762) (-5.7151, 27.7566) (-5.7551, 27.7501) (-5.798, 27.7422) (-5.8437, 27.7329) (-5.8921, 27.7219) (-5.9432, 27.7093) (-5.9969, 27.6949) (-6.0532, 27.6786) (-6.1121, 27.6603) (-6.1734, 27.6398) (-6.2372, 27.6172) (-6.3033, 27.5921) (-6.3716, 27.5647) (-6.4422, 27.5347) (-6.5149, 27.5021) (-6.5897, 27.4667) (-6.6664, 27.4285) (-6.745, 27.3874) (-6.8162, 27.3484) (-6.8611, 27.3228) (-6.8794, 27.3122) knots 0 0 0 0 0.023552 0.038904 0.056302 0.075747 0.097239 0.120778 0.146364 0.173997 0.203676 0.235403 0.269176 0.304996 0.342863 0.382777 0.424738 0.468746 0.5148 0.562902 0.61305 0.665245 0.719487 0.775776 0.834112 0.894494 0.956924 1 1 1 1
  arc A8 (-6.8794, 27.3122) -> (-6.8794, 26.6076) centre (2.0124, 26.9599) ccw
  spline S17 degree 3 poles (-6.8794, 26.6076) (-6.8611, 26.597) (-6.8428, 26.5865) (-6.8244, 26.5762) (-6.7977, 26.5613) (-6.7709, 26.5465) (-6.744, 26.5321) (-6.7179, 26.5182) (-6.6917, 26.5045) (-6.6654, 26.491) (-6.6399, 26.478) (-6.6144, 26.4653) (-6.5887, 26.4529) (-6.5639, 26.4408) (-6.5389, 26.429) (-6.5139, 26.4175) (-6.4898, 26.4064) (-6.4655, 26.3955) (-6.4412, 26.3849) (-6.4178, 26.3747) (-6.3942, 26.3647) (-6.3706, 26.3549) (-6.3479, 26.3455) (-6.3251, 26.3364) (-6.3022, 26.3275) (-6.2803, 26.3189) (-6.2583, 26.3106) (-6.2362, 26.3025) (-6.215, 26.2947) (-6.1937, 26.2871) (-6.1724, 26.2798) (-6.152, 26.2728) (-6.1316, 26.266) (-6.1111, 26.2594) (-6.0915, 26.2531) (-6.0719, 26.2469) (-6.0522, 26.241) (-6.0335, 26.2354) (-6.0147, 26.23) (-5.9959, 26.2247) (-5.978, 26.2198) (-5.9601, 26.215) (-5.9422, 26.2104) (-5.9252, 26.206) (-5.9081, 26.2018) (-5.8911, 26.1978) (-5.875, 26.194) (-5.8588, 26.1903) (-5.8427, 26.1868) (-5.8275, 26.1836) (-5.8123, 26.1805) (-5.797, 26.1775) (-5.7827, 26.1747) (-5.7684, 26.1721) (-5.7541, 26.1696) (-5.7408, 26.1673) (-5.7274, 26.1651) (-5.7141, 26.1631) (-5.7017, 26.1612) (-5.6893, 26.1594) (-5.6768, 26.1578) (-5.6654, 26.1563) (-5.654, 26.1549) (-5.6425, 26.1536) (-5.6321, 26.1524) (-5.6216, 26.1513) (-5.6111, 26.1504) (-5.6016, 26.1495) (-5.5921, 26.1487) (-5.5826, 26.148) (-5.5741, 26.1474) (-5.5656, 26.1469) (-5.5571, 26.1465) (-5.5496, 26.1461) (-5.5421, 26.1458) (-5.5346, 26.1455) (-5.5231, 26.1452) (-5.5115, 26.145) (-5.5, 26.145) knots 0 0 0 0 0.043076 0.043076 0.043076 0.105506 0.105506 0.105506 0.165888 0.165888 0.165888 0.224224 0.224224 0.224224 0.280513 0.280513 0.280513 0.334755 0.334755 0.334755 0.38695 0.38695 0.38695 0.437099 0.437099 0.437099 0.4852 0.4852 0.4852 0.531254 0.531254 0.531254 0.575262 0.575262 0.575262 0.617223 0.617223 0.617223 0.657137 0.657137 0.657137 0.695004 0.695004 0.695004 0.730824 0.730824 0.730824 0.764598 0.764598 0.764598 0.796324 0.796324 0.796324 0.826004 0.826004 0.826004 0.853636 0.853636 0.853636 0.879222 0.879222 0.879222 0.902761 0.902761 0.902761 0.924253 0.924253 0.924253 0.943699 0.943699 0.943699 0.961097 0.961097 0.961097 0.976448 0.976448 0.976448 1 1 1 1
  line L26 (-5.5, 26.145) -> (-4.55, 26.145)
  line L27 (-4.55, 29.281) -> (-4.55, 30.9108)
  line L28 (-4.55, 30.9108) -> (-5.5, 30.9108)
  spline S18 degree 3 poles (-5.5, 30.9108) (-5.5115, 30.9108) (-5.5306, 30.9105) (-5.5581, 30.9093) (-5.5836, 30.9077) (-5.6121, 30.9054) (-5.6435, 30.9022) (-5.6779, 30.898) (-5.7151, 30.8926) (-5.7551, 30.8861) (-5.798, 30.8782) (-5.8437, 30.8689) (-5.8921, 30.8579) (-5.9432, 30.8453) (-5.9969, 30.8309) (-6.0532, 30.8146) (-6.1121, 30.7963) (-6.1734, 30.7758) (-6.2372, 30.7532) (-6.3033, 30.7281) (-6.3716, 30.7007) (-6.4422, 30.6707) (-6.5149, 30.6381) (-6.5897, 30.6027) (-6.6664, 30.5645) (-6.745, 30.5234) (-6.8162, 30.4844) (-6.8611, 30.4588) (-6.8794, 30.4482) knots 0 0 0 0 0.023552 0.038904 0.056302 0.075747 0.097239 0.120778 0.146364 0.173997 0.203676 0.235403 0.269176 0.304996 0.342863 0.382777 0.424738 0.468746 0.5148 0.562902 0.61305 0.665245 0.719487 0.775776 0.834112 0.894494 0.956924 1 1 1 1
  arc A9 (-6.8794, 30.4482) -> (-6.8794, 29.7436) centre (2.0124, 30.0959) ccw
  spline S19 degree 3 poles (-6.8794, 29.7436) (-6.8611, 29.733) (-6.8428, 29.7225) (-6.8244, 29.7122) (-6.7977, 29.6973) (-6.7709, 29.6825) (-6.744, 29.6681) (-6.7179, 29.6542) (-6.6917, 29.6405) (-6.6654, 29.627) (-6.6399, 29.614) (-6.6144, 29.6013) (-6.5887, 29.5889) (-6.5639, 29.5768) (-6.5389, 29.565) (-6.5139, 29.5535) (-6.4898, 29.5424) (-6.4655, 29.5315) (-6.4412, 29.5209) (-6.4178, 29.5107) (-6.3942, 29.5007) (-6.3706, 29.4909) (-6.3479, 29.4815) (-6.3251, 29.4724) (-6.3022, 29.4635) (-6.2803, 29.4549) (-6.2583, 29.4466) (-6.2362, 29.4385) (-6.215, 29.4307) (-6.1937, 29.4231) (-6.1724, 29.4158) (-6.152, 29.4088) (-6.1316, 29.402) (-6.1111, 29.3954) (-6.0915, 29.3891) (-6.0719, 29.3829) (-6.0522, 29.377) (-6.0335, 29.3714) (-6.0147, 29.366) (-5.9959, 29.3607) (-5.978, 29.3558) (-5.9601, 29.351) (-5.9422, 29.3464) (-5.9252, 29.342) (-5.9081, 29.3378) (-5.8911, 29.3338) (-5.875, 29.33) (-5.8588, 29.3263) (-5.8427, 29.3228) (-5.8275, 29.3196) (-5.8123, 29.3165) (-5.797, 29.3135) (-5.7827, 29.3107) (-5.7684, 29.3081) (-5.7541, 29.3056) (-5.7408, 29.3033) (-5.7274, 29.3011) (-5.7141, 29.2991) (-5.7017, 29.2972) (-5.6893, 29.2954) (-5.6768, 29.2938) (-5.6654, 29.2923) (-5.654, 29.2909) (-5.6425, 29.2896) (-5.6321, 29.2884) (-5.6216, 29.2873) (-5.6111, 29.2864) (-5.6016, 29.2855) (-5.5921, 29.2847) (-5.5826, 29.284) (-5.5741, 29.2834) (-5.5656, 29.2829) (-5.5571, 29.2825) (-5.5496, 29.2821) (-5.5421, 29.2818) (-5.5346, 29.2815) (-5.5231, 29.2812) (-5.5115, 29.281) (-5.5, 29.281) knots 0 0 0 0 0.043076 0.043076 0.043076 0.105506 0.105506 0.105506 0.165888 0.165888 0.165888 0.224224 0.224224 0.224224 0.280513 0.280513 0.280513 0.334755 0.334755 0.334755 0.38695 0.38695 0.38695 0.437099 0.437099 0.437099 0.4852 0.4852 0.4852 0.531254 0.531254 0.531254 0.575262 0.575262 0.575262 0.617223 0.617223 0.617223 0.657137 0.657137 0.657137 0.695004 0.695004 0.695004 0.730824 0.730824 0.730824 0.764598 0.764598 0.764598 0.796324 0.796324 0.796324 0.826004 0.826004 0.826004 0.853636 0.853636 0.853636 0.879222 0.879222 0.879222 0.902761 0.902761 0.902761 0.924253 0.924253 0.924253 0.943699 0.943699 0.943699 0.961097 0.961097 0.961097 0.976448 0.976448 0.976448 1 1 1 1
  line L29 (-5.5, 29.281) -> (-4.55, 29.281)
  line L30 (-4.55, 32.417) -> (-4.55, 34.0468)
  line L31 (-4.55, 34.0468) -> (-5.5, 34.0468)
  spline S20 degree 3 poles (-5.5, 34.0468) (-5.5115, 34.0468) (-5.5306, 34.0465) (-5.5581, 34.0453) (-5.5836, 34.0437) (-5.6121, 34.0414) (-5.6435, 34.0382) (-5.6779, 34.034) (-5.7151, 34.0286) (-5.7551, 34.0221) (-5.798, 34.0142) (-5.8437, 34.0049) (-5.8921, 33.9939) (-5.9432, 33.9813) (-5.9969, 33.9669) (-6.0532, 33.9506) (-6.1121, 33.9323) (-6.1734, 33.9118) (-6.2372, 33.8892) (-6.3033, 33.8641) (-6.3716, 33.8367) (-6.4422, 33.8067) (-6.5149, 33.7741) (-6.5897, 33.7387) (-6.6664, 33.7005) (-6.745, 33.6594) (-6.8162, 33.6204) (-6.8611, 33.5948) (-6.8794, 33.5842) knots 0 0 0 0 0.023552 0.038904 0.056302 0.075747 0.097239 0.120778 0.146364 0.173997 0.203676 0.235403 0.269176 0.304996 0.342863 0.382777 0.424738 0.468746 0.5148 0.562902 0.61305 0.665245 0.719487 0.775776 0.834112 0.894494 0.956924 1 1 1 1
  arc A10 (-6.8794, 33.5842) -> (-6.8794, 32.8796) centre (2.0124, 33.2319) ccw
  spline S21 degree 3 poles (-6.8794, 32.8796) (-6.8611, 32.869) (-6.8428, 32.8585) (-6.8244, 32.8482) (-6.7977, 32.8333) (-6.7709, 32.8185) (-6.744, 32.8041) (-6.7179, 32.7902) (-6.6917, 32.7765) (-6.6654, 32.763) (-6.6399, 32.75) (-6.6144, 32.7373) (-6.5887, 32.7249) (-6.5639, 32.7128) (-6.5389, 32.701) (-6.5139, 32.6895) (-6.4898, 32.6784) (-6.4655, 32.6675) (-6.4412, 32.6569) (-6.4178, 32.6467) (-6.3942, 32.6367) (-6.3706, 32.6269) (-6.3479, 32.6175) (-6.3251, 32.6084) (-6.3022, 32.5995) (-6.2803, 32.5909) (-6.2583, 32.5826) (-6.2362, 32.5745) (-6.215, 32.5667) (-6.1937, 32.5591) (-6.1724, 32.5518) (-6.152, 32.5448) (-6.1316, 32.538) (-6.1111, 32.5314) (-6.0915, 32.5251) (-6.0719, 32.5189) (-6.0522, 32.513) (-6.0335, 32.5074) (-6.0147, 32.502) (-5.9959, 32.4967) (-5.978, 32.4918) (-5.9601, 32.487) (-5.9422, 32.4824) (-5.9252, 32.478) (-5.9081, 32.4738) (-5.8911, 32.4698) (-5.875, 32.466) (-5.8588, 32.4623) (-5.8427, 32.4588) (-5.8275, 32.4556) (-5.8123, 32.4525) (-5.797, 32.4495) (-5.7827, 32.4467) (-5.7684, 32.4441) (-5.7541, 32.4416) (-5.7408, 32.4393) (-5.7274, 32.4371) (-5.7141, 32.4351) (-5.7017, 32.4332) (-5.6893, 32.4314) (-5.6768, 32.4298) (-5.6654, 32.4283) (-5.654, 32.4269) (-5.6425, 32.4256) (-5.6321, 32.4244) (-5.6216, 32.4233) (-5.6111, 32.4224) (-5.6016, 32.4215) (-5.5921, 32.4207) (-5.5826, 32.42) (-5.5741, 32.4194) (-5.5656, 32.4189) (-5.5571, 32.4185) (-5.5496, 32.4181) (-5.5421, 32.4178) (-5.5346, 32.4175) (-5.5231, 32.4172) (-5.5115, 32.417) (-5.5, 32.417) knots 0 0 0 0 0.043076 0.043076 0.043076 0.105506 0.105506 0.105506 0.165888 0.165888 0.165888 0.224224 0.224224 0.224224 0.280513 0.280513 0.280513 0.334755 0.334755 0.334755 0.38695 0.38695 0.38695 0.437099 0.437099 0.437099 0.4852 0.4852 0.4852 0.531254 0.531254 0.531254 0.575262 0.575262 0.575262 0.617223 0.617223 0.617223 0.657137 0.657137 0.657137 0.695004 0.695004 0.695004 0.730824 0.730824 0.730824 0.764598 0.764598 0.764598 0.796324 0.796324 0.796324 0.826004 0.826004 0.826004 0.853636 0.853636 0.853636 0.879222 0.879222 0.879222 0.902761 0.902761 0.902761 0.924253 0.924253 0.924253 0.943699 0.943699 0.943699 0.961097 0.961097 0.961097 0.976448 0.976448 0.976448 1 1 1 1
  line L32 (-5.5, 32.417) -> (-4.55, 32.417)
  line L33 (-4.55, 35.553) -> (-4.55, 37.1828)
  line L34 (-4.55, 37.1828) -> (-5.5, 37.1828)
  spline S22 degree 3 poles (-5.5, 37.1828) (-5.5115, 37.1828) (-5.5306, 37.1825) (-5.5581, 37.1813) (-5.5836, 37.1797) (-5.6121, 37.1774) (-5.6435, 37.1742) (-5.6779, 37.17) (-5.7151, 37.1646) (-5.7551, 37.1581) (-5.798, 37.1502) (-5.8437, 37.1409) (-5.8921, 37.1299) (-5.9432, 37.1173) (-5.9969, 37.1029) (-6.0532, 37.0866) (-6.1121, 37.0683) (-6.1734, 37.0478) (-6.2372, 37.0252) (-6.3033, 37.0001) (-6.3716, 36.9727) (-6.4422, 36.9427) (-6.5149, 36.9101) (-6.5897, 36.8747) (-6.6664, 36.8365) (-6.745, 36.7954) (-6.8162, 36.7564) (-6.8611, 36.7308) (-6.8794, 36.7202) knots 0 0 0 0 0.023552 0.038904 0.056302 0.075747 0.097239 0.120778 0.146364 0.173997 0.203676 0.235403 0.269176 0.304996 0.342863 0.382777 0.424738 0.468746 0.5148 0.562902 0.61305 0.665245 0.719487 0.775776 0.834112 0.894494 0.956924 1 1 1 1
  arc A11 (-6.8794, 36.7202) -> (-6.8794, 36.0156) centre (2.0124, 36.3679) ccw
  spline S23 degree 3 poles (-6.8794, 36.0156) (-6.8611, 36.005) (-6.8428, 35.9945) (-6.8244, 35.9842) (-6.7977, 35.9693) (-6.7709, 35.9545) (-6.744, 35.9401) (-6.7179, 35.9262) (-6.6917, 35.9125) (-6.6654, 35.899) (-6.6399, 35.886) (-6.6144, 35.8733) (-6.5887, 35.8609) (-6.5639, 35.8488) (-6.5389, 35.837) (-6.5139, 35.8255) (-6.4898, 35.8144) (-6.4655, 35.8035) (-6.4412, 35.7929) (-6.4178, 35.7827) (-6.3942, 35.7727) (-6.3706, 35.7629) (-6.3479, 35.7535) (-6.3251, 35.7444) (-6.3022, 35.7355) (-6.2803, 35.7269) (-6.2583, 35.7186) (-6.2362, 35.7105) (-6.215, 35.7027) (-6.1937, 35.6951) (-6.1724, 35.6878) (-6.152, 35.6808) (-6.1316, 35.674) (-6.1111, 35.6674) (-6.0915, 35.6611) (-6.0719, 35.6549) (-6.0522, 35.649) (-6.0335, 35.6434) (-6.0147, 35.638) (-5.9959, 35.6327) (-5.978, 35.6278) (-5.9601, 35.623) (-5.9422, 35.6184) (-5.9252, 35.614) (-5.9081, 35.6098) (-5.8911, 35.6058) (-5.875, 35.602) (-5.8588, 35.5983) (-5.8427, 35.5948) (-5.8275, 35.5916) (-5.8123, 35.5885) (-5.797, 35.5855) (-5.7827, 35.5827) (-5.7684, 35.5801) (-5.7541, 35.5776) (-5.7408, 35.5753) (-5.7274, 35.5731) (-5.7141, 35.5711) (-5.7017, 35.5692) (-5.6893, 35.5674) (-5.6768, 35.5658) (-5.6654, 35.5643) (-5.654, 35.5629) (-5.6425, 35.5616) (-5.6321, 35.5604) (-5.6216, 35.5593) (-5.6111, 35.5584) (-5.6016, 35.5575) (-5.5921, 35.5567) (-5.5826, 35.556) (-5.5741, 35.5554) (-5.5656, 35.5549) (-5.5571, 35.5545) (-5.5496, 35.5541) (-5.5421, 35.5538) (-5.5346, 35.5535) (-5.5231, 35.5532) (-5.5115, 35.553) (-5.5, 35.553) knots 0 0 0 0 0.043076 0.043076 0.043076 0.105506 0.105506 0.105506 0.165888 0.165888 0.165888 0.224224 0.224224 0.224224 0.280513 0.280513 0.280513 0.334755 0.334755 0.334755 0.38695 0.38695 0.38695 0.437099 0.437099 0.437099 0.4852 0.4852 0.4852 0.531254 0.531254 0.531254 0.575262 0.575262 0.575262 0.617223 0.617223 0.617223 0.657137 0.657137 0.657137 0.695004 0.695004 0.695004 0.730824 0.730824 0.730824 0.764598 0.764598 0.764598 0.796324 0.796324 0.796324 0.826004 0.826004 0.826004 0.853636 0.853636 0.853636 0.879222 0.879222 0.879222 0.902761 0.902761 0.902761 0.924253 0.924253 0.924253 0.943699 0.943699 0.943699 0.961097 0.961097 0.961097 0.976448 0.976448 0.976448 1 1 1 1
  line L35 (-5.5, 35.553) -> (-4.55, 35.553)
  line L36 (-4.55, 38.689) -> (-4.55, 40.3188)
  line L37 (-4.55, 40.3188) -> (-5.5, 40.3188)
  spline S24 degree 3 poles (-5.5, 40.3188) (-5.5115, 40.3188) (-5.5306, 40.3185) (-5.5581, 40.3173) (-5.5836, 40.3157) (-5.6121, 40.3134) (-5.6435, 40.3102) (-5.6779, 40.306) (-5.7151, 40.3006) (-5.7551, 40.2941) (-5.798, 40.2862) (-5.8437, 40.2769) (-5.8921, 40.2659) (-5.9432, 40.2533) (-5.9969, 40.2389) (-6.0532, 40.2226) (-6.1121, 40.2043) (-6.1734, 40.1838) (-6.2372, 40.1612) (-6.3033, 40.1361) (-6.3716, 40.1087) (-6.4422, 40.0787) (-6.5149, 40.0461) (-6.5897, 40.0107) (-6.6664, 39.9725) (-6.745, 39.9314) (-6.8162, 39.8924) (-6.8611, 39.8668) (-6.8794, 39.8562) knots 0 0 0 0 0.023552 0.038904 0.056302 0.075747 0.097239 0.120778 0.146364 0.173997 0.203676 0.235403 0.269176 0.304996 0.342863 0.382777 0.424738 0.468746 0.5148 0.562902 0.61305 0.665245 0.719487 0.775776 0.834112 0.894494 0.956924 1 1 1 1
  arc A12 (-6.8794, 39.8562) -> (-6.8794, 39.1516) centre (2.0124, 39.5039) ccw
  spline S25 degree 3 poles (-6.8794, 39.1516) (-6.8611, 39.141) (-6.8428, 39.1305) (-6.8244, 39.1202) (-6.7977, 39.1053) (-6.7709, 39.0905) (-6.744, 39.0761) (-6.7179, 39.0622) (-6.6917, 39.0485) (-6.6654, 39.035) (-6.6399, 39.022) (-6.6144, 39.0093) (-6.5887, 38.9969) (-6.5639, 38.9848) (-6.5389, 38.973) (-6.5139, 38.9615) (-6.4898, 38.9504) (-6.4655, 38.9395) (-6.4412, 38.9289) (-6.4178, 38.9187) (-6.3942, 38.9087) (-6.3706, 38.8989) (-6.3479, 38.8895) (-6.3251, 38.8804) (-6.3022, 38.8715) (-6.2803, 38.8629) (-6.2583, 38.8546) (-6.2362, 38.8465) (-6.215, 38.8387) (-6.1937, 38.8311) (-6.1724, 38.8238) (-6.152, 38.8168) (-6.1316, 38.81) (-6.1111, 38.8034) (-6.0915, 38.7971) (-6.0719, 38.7909) (-6.0522, 38.785) (-6.0335, 38.7794) (-6.0147, 38.774) (-5.9959, 38.7687) (-5.978, 38.7638) (-5.9601, 38.759) (-5.9422, 38.7544) (-5.9252, 38.75) (-5.9081, 38.7458) (-5.8911, 38.7418) (-5.875, 38.738) (-5.8588, 38.7343) (-5.8427, 38.7308) (-5.8275, 38.7276) (-5.8123, 38.7245) (-5.797, 38.7215) (-5.7827, 38.7187) (-5.7684, 38.7161) (-5.7541, 38.7136) (-5.7408, 38.7113) (-5.7274, 38.7091) (-5.7141, 38.7071) (-5.7017, 38.7052) (-5.6893, 38.7034) (-5.6768, 38.7018) (-5.6654, 38.7003) (-5.654, 38.6989) (-5.6425, 38.6976) (-5.6321, 38.6964) (-5.6216, 38.6953) (-5.6111, 38.6944) (-5.6016, 38.6935) (-5.5921, 38.6927) (-5.5826, 38.692) (-5.5741, 38.6914) (-5.5656, 38.6909) (-5.5571, 38.6905) (-5.5496, 38.6901) (-5.5421, 38.6898) (-5.5346, 38.6895) (-5.5231, 38.6892) (-5.5115, 38.689) (-5.5, 38.689) knots 0 0 0 0 0.043076 0.043076 0.043076 0.105506 0.105506 0.105506 0.165888 0.165888 0.165888 0.224224 0.224224 0.224224 0.280513 0.280513 0.280513 0.334755 0.334755 0.334755 0.38695 0.38695 0.38695 0.437099 0.437099 0.437099 0.4852 0.4852 0.4852 0.531254 0.531254 0.531254 0.575262 0.575262 0.575262 0.617223 0.617223 0.617223 0.657137 0.657137 0.657137 0.695004 0.695004 0.695004 0.730824 0.730824 0.730824 0.764598 0.764598 0.764598 0.796324 0.796324 0.796324 0.826004 0.826004 0.826004 0.853636 0.853636 0.853636 0.879222 0.879222 0.879222 0.902761 0.902761 0.902761 0.924253 0.924253 0.924253 0.943699 0.943699 0.943699 0.961097 0.961097 0.961097 0.976448 0.976448 0.976448 1 1 1 1
  line L38 (-5.5, 38.689) -> (-4.55, 38.689)
  line L39 (-4.55, 41.825) -> (-4.55, 43.4548)
  line L40 (-4.55, 43.4548) -> (-5.5, 43.4548)
  spline S26 degree 3 poles (-5.5, 43.4548) (-5.5115, 43.4548) (-5.5306, 43.4545) (-5.5581, 43.4533) (-5.5836, 43.4517) (-5.6121, 43.4494) (-5.6435, 43.4462) (-5.6779, 43.442) (-5.7151, 43.4366) (-5.7551, 43.4301) (-5.798, 43.4222) (-5.8437, 43.4129) (-5.8921, 43.4019) (-5.9432, 43.3893) (-5.9969, 43.3749) (-6.0532, 43.3586) (-6.1121, 43.3403) (-6.1734, 43.3198) (-6.2372, 43.2972) (-6.3033, 43.2721) (-6.3716, 43.2447) (-6.4422, 43.2147) (-6.5149, 43.1821) (-6.5897, 43.1467) (-6.6664, 43.1085) (-6.745, 43.0674) (-6.8162, 43.0284) (-6.8611, 43.0028) (-6.8794, 42.9922) knots 0 0 0 0 0.023552 0.038904 0.056302 0.075747 0.097239 0.120778 0.146364 0.173997 0.203676 0.235403 0.269176 0.304996 0.342863 0.382777 0.424738 0.468746 0.5148 0.562902 0.61305 0.665245 0.719487 0.775776 0.834112 0.894494 0.956924 1 1 1 1
  arc A13 (-6.8794, 42.9922) -> (-6.8794, 42.2876) centre (2.0124, 42.6399) ccw